Autodesk Fusion 360 part; units mm, degrees
(part 6 of 8)
  spline S180 degree 3 poles (738.6544, -32.0173) (738.4476, -32.017) (738.2428, -32.0571) (737.8602, -32.2135) (737.6859, -32.3284) (737.4231, -32.587) (737.3257, -32.7177) (737.1739, -33.004) (737.1203, -33.1579) (737.0909, -33.3172) knots 0 0 0 0 0.062015 0.062015 0.12403 0.12403 0.172638 0.172638 0.221247 0.221247 0.221247 0.221247
  spline S181 degree 5 poles (738.6544, -32.0173) (738.6823, -32.0173) (738.802, -32.0174) (739.0135, -32.0169) (739.317, -32.0149) (739.7125, -32.0096) (740.1723, -31.9999) (740.6323, -31.9868) (741.0925, -31.9701) (741.553, -31.9499) (742.0138, -31.9262) (742.4748, -31.8993) (742.9359, -31.8692) (743.3973, -31.8361) (743.8588, -31.8) (744.3204, -31.7611) (744.7821, -31.7194) (745.2439, -31.6749) (745.7059, -31.6277) (746.1679, -31.5778) (746.63, -31.5252) (747.0922, -31.47) (747.5544, -31.4123) (748.0167, -31.3521) (748.4791, -31.2893) (748.9414, -31.2242) (749.4038, -31.1567) (749.8663, -31.0868) (750.3287, -31.0146) (750.7911, -30.94) (751.2535, -30.8632) (751.716, -30.7841) (752.1784, -30.7028) (752.6408, -30.6193) (753.1031, -30.5336) (753.5654, -30.4458) (754.0277, -30.3558) (754.4899, -30.2638) (754.9521, -30.1696) (755.4142, -30.0734) (755.8763, -29.9751) (756.3382, -29.8748) (756.8001, -29.7725) (757.262, -29.6682) (757.7237, -29.5619) (758.1854, -29.4537) (758.6469, -29.3435) (759.1084, -29.2314) (759.5698, -29.1173) (760.031, -29.0014) (760.4922, -28.8836) (760.9532, -28.764) (761.4141, -28.6424) (761.8749, -28.5191) (762.3356, -28.3939) (762.7961, -28.2668) (763.2565, -28.138) (763.7168, -28.0074) (764.1769, -27.8751) (764.6368, -27.7409) (765.0966, -27.605) (765.5563, -27.4674) (765.9239, -27.3558) (766.1995, -27.2714) (766.3832, -27.2148) (766.4751, -27.1864) knots 0.13851185 0.13851185 0.13851185 0.13851185 0.13851185 0.13851185 0.14285714 0.15714286 0.17142857 0.18571429 0.2 0.21428571 0.22857143 0.24285714 0.25714286 0.27142857 0.28571429 0.3 0.31428571 0.32857143 0.34285714 0.35714286 0.37142857 0.38571429 0.4 0.41428571 0.42857143 0.44285714 0.45714286 0.47142857 0.48571429 0.5 0.51428571 0.52857143 0.54285714 0.55714286 0.57142857 0.58571429 0.6 0.61428571 0.62857143 0.64285714 0.65714286 0.67142857 0.68571429 0.7 0.71428571 0.72857143 0.74285714 0.75714286 0.77142857 0.78571429 0.8 0.81428571 0.82857143 0.84285714 0.85714286 0.87142857 0.88571429 0.9 0.91428571 0.92857143 0.94285714 0.95714286 0.97142857 0.98571429 1 1 1 1 1 1
  arc A91 (766.4751, -27.1864) -> (767.7563, -17.4547) centre (452.3696, 19.1166) ccw
  spline S182 degree 5 poles (767.7563, -17.4547) (767.6749, -17.4034) (767.5121, -17.3012) (767.2677, -17.1483) (766.9415, -16.9455) (766.5331, -16.6935) (766.1242, -16.4433) (765.7146, -16.1946) (765.3045, -15.9477) (764.8937, -15.7024) (764.4823, -15.4588) (764.0704, -15.217) (763.6578, -14.9768) (763.2446, -14.7384) (762.8309, -14.5017) (762.4165, -14.2668) (762.0016, -14.0336) (761.586, -13.8023) (761.1699, -13.5727) (760.7532, -13.345) (760.3359, -13.1191) (759.918, -12.8951) (759.4994, -12.6729) (759.0803, -12.4526) (758.6607, -12.2343) (758.2404, -12.0178) (757.8195, -11.8033) (757.398, -11.5907) (756.976, -11.3802) (756.5533, -11.1716) (756.1301, -10.9651) (755.7063, -10.7606) (755.2819, -10.5581) (754.8568, -10.3578) (754.4312, -10.1596) (754.005, -9.9635) (753.5783, -9.7696) (753.1509, -9.5779) (752.7229, -9.3885) (752.2943, -9.2013) (751.8652, -9.0164) (751.4354, -8.8338) (751.005, -8.6536) (750.5741, -8.4757) (750.1425, -8.3003) (749.7104, -8.1274) (749.2776, -7.957) (748.8443, -7.7892) (748.4103, -7.624) (747.9757, -7.4616) (747.5405, -7.3018) (747.1047, -7.1447) (746.6683, -6.9904) (746.2312, -6.839) (745.7936, -6.6906) (745.3553, -6.5453) (744.9163, -6.4032) (744.4767, -6.2645) (744.0365, -6.1292) (743.5955, -5.9975) (743.154, -5.8692) (742.7733, -5.7617) (742.4807, -5.6811) (742.2765, -5.626) (742.1608, -5.5951) (742.1339, -5.5879) knots -1 -1 -1 -1 -1 -1 -0.98571429 -0.97142857 -0.95714286 -0.94285714 -0.92857143 -0.91428571 -0.9 -0.88571429 -0.87142857 -0.85714286 -0.84285714 -0.82857143 -0.81428571 -0.8 -0.78571429 -0.77142857 -0.75714286 -0.74285714 -0.72857143 -0.71428571 -0.7 -0.68571429 -0.67142857 -0.65714286 -0.64285714 -0.62857143 -0.61428571 -0.6 -0.58571429 -0.57142857 -0.55714286 -0.54285714 -0.52857143 -0.51428571 -0.5 -0.48571429 -0.47142857 -0.45714286 -0.44285714 -0.42857143 -0.41428571 -0.4 -0.38571429 -0.37142857 -0.35714286 -0.34285714 -0.32857143 -0.31428571 -0.3 -0.28571429 -0.27142857 -0.25714286 -0.24285714 -0.22857143 -0.21428571 -0.2 -0.18571429 -0.17142857 -0.15714286 -0.14285714 -0.13851185 -0.13851185 -0.13851185 -0.13851185 -0.13851185 -0.13851185
  spline S183 degree 3 poles (740.9602, -3.9275) (740.9437, -4.1336) (740.9677, -4.3409) (741.0937, -4.7347) (741.1945, -4.9173) (741.4319, -5.1996) (741.5545, -5.3069) (741.828, -5.4807) (741.9773, -5.5461) (742.1339, -5.5879) knots 0 0 0 0 0.062015 0.062015 0.12403 0.12403 0.172638 0.172638 0.221247 0.221247 0.221247 0.221247
  arc A92 (740.9602, -3.9275) -> (741.4991, 4.2949) centre (452.3696, 19.1166) ccw
  spline S184 degree 3 poles (742.8795, 5.7879) (742.6745, 5.7612) (742.4767, 5.6947) (742.1177, 5.4896) (741.9599, 5.353) (741.7331, 5.0623) (741.6536, 4.92) (741.5404, 4.6163) (741.5074, 4.4567) (741.4991, 4.2949) knots 0 0 0 0 0.062015 0.062015 0.12403 0.12403 0.172638 0.172638 0.221247 0.221247 0.221247 0.221247
  spline S185 degree 5 poles (742.8795, 5.7879) (742.9071, 5.7915) (743.0258, 5.807) (743.2355, 5.8351) (743.5361, 5.8767) (743.9276, 5.9336) (744.3821, 6.0032) (744.8364, 6.0763) (745.2906, 6.1529) (745.7445, 6.233) (746.1983, 6.3166) (746.6518, 6.4035) (747.1051, 6.4935) (747.5582, 6.5866) (748.011, 6.6826) (748.4636, 6.7814) (748.9159, 6.883) (749.368, 6.9874) (749.8198, 7.0945) (750.2713, 7.2043) (750.7226, 7.3167) (751.1737, 7.4318) (751.6244, 7.5493) (752.0749, 7.6694) (752.5251, 7.7919) (752.975, 7.9169) (753.4247, 8.0442) (753.874, 8.1738) (754.323, 8.3058) (754.7718, 8.4401) (755.2202, 8.5766) (755.6684, 8.7153) (756.1162, 8.8563) (756.5637, 8.9995) (757.0109, 9.1448) (757.4578, 9.2922) (757.9044, 9.4417) (758.3507, 9.5933) (758.7966, 9.747) (759.2422, 9.9027) (759.6875, 10.0605) (760.1324, 10.2202) (760.577, 10.3819) (761.0213, 10.5456) (761.4652, 10.7113) (761.9088, 10.8788) (762.352, 11.0483) (762.7949, 11.2197) (763.2374, 11.393) (763.6796, 11.5681) (764.1214, 11.7451) (764.5629, 11.9239) (765.004, 12.1046) (765.4448, 12.287) (765.8851, 12.4713) (766.3252, 12.6573) (766.7648, 12.8451) (767.2041, 13.0347) (767.6429, 13.226) (768.0815, 13.419) (768.5196, 13.6138) (768.9573, 13.8102) (769.3072, 13.9688) (769.5695, 14.0885) (769.7443, 14.1686) (769.8316, 14.2087) knots 0.13851185 0.13851185 0.13851185 0.13851185 0.13851185 0.13851185 0.14285714 0.15714286 0.17142857 0.18571429 0.2 0.21428571 0.22857143 0.24285714 0.25714286 0.27142857 0.28571429 0.3 0.31428571 0.32857143 0.34285714 0.35714286 0.37142857 0.38571429 0.4 0.41428571 0.42857143 0.44285714 0.45714286 0.47142857 0.48571429 0.5 0.51428571 0.52857143 0.54285714 0.55714286 0.57142857 0.58571429 0.6 0.61428571 0.62857143 0.64285714 0.65714286 0.67142857 0.68571429 0.7 0.71428571 0.72857143 0.74285714 0.75714286 0.77142857 0.78571429 0.8 0.81428571 0.82857143 0.84285714 0.85714286 0.87142857 0.88571429 0.9 0.91428571 0.92857143 0.94285714 0.95714286 0.97142857 0.98571429 1 1 1 1 1 1
  arc A93 (769.8316, 14.2087) -> (769.8316, 24.0244) centre (452.3696, 19.1166) ccw
  spline S186 degree 5 poles (769.8316, 24.0244) (769.7443, 24.0646) (769.5695, 24.1447) (769.3072, 24.2644) (768.9573, 24.4229) (768.5196, 24.6194) (768.0815, 24.8142) (767.6429, 25.0072) (767.2041, 25.1985) (766.7648, 25.388) (766.3252, 25.5759) (765.8851, 25.7619) (765.4448, 25.9461) (765.004, 26.1286) (764.5629, 26.3093) (764.1214, 26.4881) (763.6796, 26.6651) (763.2374, 26.8402) (762.7949, 27.0135) (762.352, 27.1848) (761.9088, 27.3543) (761.4652, 27.5219) (761.0213, 27.6875) (760.577, 27.8512) (760.1324, 28.013) (759.6875, 28.1727) (759.2422, 28.3305) (758.7966, 28.4862) (758.3507, 28.6399) (757.9044, 28.7915) (757.4578, 28.941) (757.0109, 29.0884) (756.5637, 29.2337) (756.1162, 29.3769) (755.6684, 29.5178) (755.2202, 29.6566) (754.7718, 29.7931) (754.323, 29.9274) (753.874, 30.0594) (753.4247, 30.189) (752.975, 30.3163) (752.5251, 30.4412) (752.0749, 30.5638) (751.6244, 30.6838) (751.1737, 30.8014) (750.7226, 30.9165) (750.2713, 31.0289) (749.8198, 31.1387) (749.368, 31.2458) (748.9159, 31.3502) (748.4636, 31.4518) (748.011, 31.5506) (747.5582, 31.6466) (747.1051, 31.7397) (746.6518, 31.8297) (746.1983, 31.9166) (745.7445, 32.0001) (745.2906, 32.0803) (744.8364, 32.1569) (744.3821, 32.23) (743.9276, 32.2996) (743.5361, 32.3564) (743.2355, 32.3981) (743.0258, 32.4262) (742.9071, 32.4417) (742.8795, 32.4453) knots -1 -1 -1 -1 -1 -1 -0.98571429 -0.97142857 -0.95714286 -0.94285714 -0.92857143 -0.91428571 -0.9 -0.88571429 -0.87142857 -0.85714286 -0.84285714 -0.82857143 -0.81428571 -0.8 -0.78571429 -0.77142857 -0.75714286 -0.74285714 -0.72857143 -0.71428571 -0.7 -0.68571429 -0.67142857 -0.65714286 -0.64285714 -0.62857143 -0.61428571 -0.6 -0.58571429 -0.57142857 -0.55714286 -0.54285714 -0.52857143 -0.51428571 -0.5 -0.48571429 -0.47142857 -0.45714286 -0.44285714 -0.42857143 -0.41428571 -0.4 -0.38571429 -0.37142857 -0.35714286 -0.34285714 -0.32857143 -0.31428571 -0.3 -0.28571429 -0.27142857 -0.25714286 -0.24285714 -0.22857143 -0.21428571 -0.2 -0.18571429 -0.17142857 -0.15714286 -0.14285714 -0.13851185 -0.13851185 -0.13851185 -0.13851185 -0.13851185 -0.13851185
  spline S187 degree 3 poles (741.4991, 33.9382) (741.5097, 33.7318) (741.5605, 33.5294) (741.7368, 33.1555) (741.8607, 32.9875) (742.1328, 32.7387) (742.2684, 32.6483) (742.5623, 32.5117) (742.7188, 32.4662) (742.8795, 32.4453) knots 0 0 0 0 0.062015 0.062015 0.12403 0.12403 0.172638 0.172638 0.221247 0.221247 0.221247 0.221247
  arc A94 (741.4991, 33.9382) -> (740.9602, 42.1607) centre (452.3696, 19.1166) ccw
  spline S188 degree 3 poles (742.1339, 43.821) (741.9341, 43.7678) (741.7467, 43.6761) (741.4175, 43.4259) (741.2789, 43.2699) (741.092, 42.952) (741.0318, 42.8006) (740.9592, 42.4848) (740.9473, 42.3222) (740.9602, 42.1607) knots 0 0 0 0 0.062015 0.062015 0.12403 0.12403 0.172638 0.172638 0.221247 0.221247 0.221247 0.221247
  spline S189 degree 5 poles (742.1339, 43.821) (742.1608, 43.8282) (742.2765, 43.8591) (742.4807, 43.9143) (742.7733, 43.9949) (743.154, 44.1023) (743.5955, 44.2306) (744.0365, 44.3624) (744.4767, 44.4977) (744.9163, 44.6364) (745.3553, 44.7784) (745.7936, 44.9238) (746.2312, 45.0722) (746.6683, 45.2236) (747.1047, 45.3779) (747.5405, 45.5349) (747.9757, 45.6947) (748.4103, 45.8572) (748.8443, 46.0224) (749.2776, 46.1902) (749.7104, 46.3606) (750.1425, 46.5335) (750.5741, 46.7089) (751.005, 46.8867) (751.4354, 47.067) (751.8652, 47.2496) (752.2943, 47.4345) (752.7229, 47.6217) (753.1509, 47.8111) (753.5783, 48.0028) (754.005, 48.1967) (754.4312, 48.3928) (754.8568, 48.591) (755.2819, 48.7913) (755.7063, 48.9937) (756.1301, 49.1982) (756.5533, 49.4048) (756.976, 49.6133) (757.398, 49.8239) (757.8195, 50.0365) (758.2404, 50.251) (758.6607, 50.4674) (759.0803, 50.6858) (759.4994, 50.9061) (759.918, 51.1283) (760.3359, 51.3523) (760.7532, 51.5782) (761.1699, 51.8059) (761.586, 52.0355) (762.0016, 52.2668) (762.4165, 52.4999) (762.8309, 52.7349) (763.2446, 52.9715) (763.6578, 53.21) (764.0704, 53.4501) (764.4823, 53.692) (764.8937, 53.9356) (765.3045, 54.1809) (765.7146, 54.4278) (766.1242, 54.6764) (766.5331, 54.9267) (766.9415, 55.1786) (767.2677, 55.3815) (767.5121, 55.5344) (767.6749, 55.6366) (767.7563, 55.6878) knots 0.13851185 0.13851185 0.13851185 0.13851185 0.13851185 0.13851185 0.14285714 0.15714286 0.17142857 0.18571429 0.2 0.21428571 0.22857143 0.24285714 0.25714286 0.27142857 0.28571429 0.3 0.31428571 0.32857143 0.34285714 0.35714286 0.37142857 0.38571429 0.4 0.41428571 0.42857143 0.44285714 0.45714286 0.47142857 0.48571429 0.5 0.51428571 0.52857143 0.54285714 0.55714286 0.57142857 0.58571429 0.6 0.61428571 0.62857143 0.64285714 0.65714286 0.67142857 0.68571429 0.7 0.71428571 0.72857143 0.74285714 0.75714286 0.77142857 0.78571429 0.8 0.81428571 0.82857143 0.84285714 0.85714286 0.87142857 0.88571429 0.9 0.91428571 0.92857143 0.94285714 0.95714286 0.97142857 0.98571429 1 1 1 1 1 1
  arc A95 (767.7563, 55.6878) -> (766.4751, 65.4196) centre (452.3696, 19.1166) ccw
  spline S190 degree 5 poles (766.4751, 65.4196) (766.3832, 65.448) (766.1995, 65.5046) (765.9239, 65.589) (765.5563, 65.7005) (765.0966, 65.8382) (764.6368, 65.9741) (764.1769, 66.1082) (763.7168, 66.2406) (763.2565, 66.3712) (762.7961, 66.5) (762.3356, 66.627) (761.8749, 66.7522) (761.4141, 66.8756) (760.9532, 66.9971) (760.4922, 67.1168) (760.031, 67.2346) (759.5698, 67.3505) (759.1084, 67.4645) (758.6469, 67.5766) (758.1854, 67.6868) (757.7237, 67.7951) (757.262, 67.9014) (756.8001, 68.0057) (756.3382, 68.108) (755.8763, 68.2083) (755.4142, 68.3065) (754.9521, 68.4028) (754.4899, 68.4969) (754.0277, 68.589) (753.5654, 68.679) (753.1031, 68.7668) (752.6408, 68.8525) (752.1784, 68.936) (751.716, 69.0173) (751.2535, 69.0964) (750.7911, 69.1732) (750.3287, 69.2477) (749.8663, 69.32) (749.4038, 69.3899) (748.9414, 69.4574) (748.4791, 69.5225) (748.0167, 69.5852) (747.5544, 69.6455) (747.0922, 69.7032) (746.63, 69.7584) (746.1679, 69.811) (745.7059, 69.8609) (745.2439, 69.9081) (744.7821, 69.9526) (744.3204, 69.9943) (743.8588, 70.0332) (743.3973, 70.0692) (742.9359, 70.1024) (742.4748, 70.1325) (742.0138, 70.1594) (741.553, 70.183) (741.0925, 70.2032) (740.6323, 70.2199) (740.1723, 70.2331) (739.7125, 70.2428) (739.317, 70.248) (739.0135, 70.2501) (738.802, 70.2506) (738.6823, 70.2505) (738.6544, 70.2504) knots -1 -1 -1 -1 -1 -1 -0.98571429 -0.97142857 -0.95714286 -0.94285714 -0.92857143 -0.91428571 -0.9 -0.88571429 -0.87142857 -0.85714286 -0.84285714 -0.82857143 -0.81428571 -0.8 -0.78571429 -0.77142857 -0.75714286 -0.74285714 -0.72857143 -0.71428571 -0.7 -0.68571429 -0.67142857 -0.65714286 -0.64285714 -0.62857143 -0.61428571 -0.6 -0.58571429 -0.57142857 -0.55714286 -0.54285714 -0.52857143 -0.51428571 -0.5 -0.48571429 -0.47142857 -0.45714286 -0.44285714 -0.42857143 -0.41428571 -0.4 -0.38571429 -0.37142857 -0.35714286 -0.34285714 -0.32857143 -0.31428571 -0.3 -0.28571429 -0.27142857 -0.25714286 -0.24285714 -0.22857143 -0.21428571 -0.2 -0.18571429 -0.17142857 -0.15714286 -0.14285714 -0.13851185 -0.13851185 -0.13851185 -0.13851185 -0.13851185 -0.13851185
  spline S191 degree 3 poles (737.0909, 71.5504) (737.1284, 71.3471) (737.2052, 71.1531) (737.4288, 70.8054) (737.5735, 70.655) (737.8758, 70.4438) (738.022, 70.3719) (738.3312, 70.2748) (738.4923, 70.2502) (738.6544, 70.2504) knots 0 0 0 0 0.062015 0.062015 0.12403 0.12403 0.172638 0.172638 0.221247 0.221247 0.221247 0.221247
  circle A96 centre (452.3696, 19.1166) radius 12.7
  circle A97 centre (452.3696, 19.1166) radius 12.7
  dimension "d17" = 25.4
  constraint concentric A0 A97
  measures "d17" diameter of A97
extrude "Extrude1''" add sketch "Sketch1 (3)" along normal mid plane 152.4 separate body contours A96 A97 makes body 3 in component "Component"
sketch "Sketch2 (3)" plane through (0, 0, 12.7) normal (0, 0, 1) x (1, 0, 0)
  arc A0 (126.3672, -24.5983) -> (127.7662, -13.9721) centre (-8.7656, -1.4025) ccw
  arc A1 (129.4742, -12.5352) -> (127.7662, -13.9721) centre (129.347, -14.1176) ccw
  line L0 (129.4742, -12.5352) -> (133.9814, -12.8976)
  spline S0 degree 5 poles (133.9814, -12.8976) (134.0461, -12.9028) (134.1756, -12.9115) (134.3698, -12.9198) (134.629, -12.9214) (134.9532, -12.9107) (135.2776, -12.8908) (135.6022, -12.8653) (135.9267, -12.8368) (136.2513, -12.8063) (136.5759, -12.7736) (136.9004, -12.738) (137.2248, -12.6986) (137.5492, -12.6547) (137.8735, -12.6064) (138.1976, -12.5541) (138.5217, -12.4982) (138.8456, -12.4395) (139.1694, -12.3782) (139.493, -12.3146) (139.8164, -12.2485) (140.1397, -12.1799) (140.4628, -12.1087) (140.7857, -12.0347) (141.1085, -11.958) (141.431, -11.8787) (141.7533, -11.797) (142.0754, -11.713) (142.3973, -11.6267) (142.719, -11.5383) (143.0404, -11.4476) (143.3616, -11.3548) (143.6826, -11.2599) (144.0033, -11.1627) (144.3237, -11.0635) (144.6439, -10.9621) (144.9639, -10.8587) (145.2835, -10.7533) (145.6029, -10.6459) (145.922, -10.5366) (146.2409, -10.4253) (146.5594, -10.3121) (146.8777, -10.1971) (147.1957, -10.0801) (147.5133, -9.9613) (147.8307, -9.8407) (148.1478, -9.7182) (148.4645, -9.5939) (148.781, -9.4679) (149.0971, -9.3401) (149.4129, -9.2105) (149.7284, -9.0792) (150.0435, -8.9462) (150.3583, -8.8115) (150.6728, -8.6752) (150.9869, -8.5371) (151.3007, -8.3974) (151.6142, -8.256) (151.9273, -8.113) (152.24, -7.9684) (152.5524, -7.8221) (152.8644, -7.6743) (153.1761, -7.5249) (153.4874, -7.3739) (153.7983, -7.2214) (154.1088, -7.0673) (154.419, -6.9116) (154.7288, -6.7545) (155.0382, -6.5958) (155.3472, -6.4356) (155.6559, -6.2739) (155.9024, -6.1434) (156.0872, -6.0448) (156.2103, -5.9788) (156.2719, -5.9457) knots 0 0 0 0 0 0 0.01428571 0.02857143 0.04285714 0.05714286 0.07142857 0.08571429 0.1 0.11428571 0.12857143 0.14285714 0.15714286 0.17142857 0.18571429 0.2 0.21428571 0.22857143 0.24285714 0.25714286 0.27142857 0.28571429 0.3 0.31428571 0.32857143 0.34285714 0.35714286 0.37142857 0.38571429 0.4 0.41428571 0.42857143 0.44285714 0.45714286 0.47142857 0.48571429 0.5 0.51428571 0.52857143 0.54285714 0.55714286 0.57142857 0.58571429 0.6 0.61428571 0.62857143 0.64285714 0.65714286 0.67142857 0.68571429 0.7 0.71428571 0.72857143 0.74285714 0.75714286 0.77142857 0.78571429 0.8 0.81428571 0.82857143 0.84285714 0.85714286 0.87142857 0.88571429 0.9 0.91428571 0.92857143 0.94285714 0.95714286 0.97142857 0.98571429 1 1 1 1 1 1
  arc A2 (156.2719, -5.9457) -> (156.2719, 3.1407) centre (-8.7656, -1.4025) ccw
  spline S1 degree 5 poles (156.2719, 3.1407) (156.2103, 3.1738) (156.0872, 3.2398) (155.9024, 3.3384) (155.6559, 3.4689) (155.3472, 3.6306) (155.0382, 3.7908) (154.7288, 3.9495) (154.419, 4.1066) (154.1088, 4.2623) (153.7983, 4.4164) (153.4874, 4.5689) (153.1761, 4.7199) (152.8644, 4.8693) (152.5524, 5.0171) (152.24, 5.1634) (151.9273, 5.308) (151.6142, 5.451) (151.3007, 5.5924) (150.9869, 5.7321) (150.6728, 5.8702) (150.3583, 6.0065) (150.0435, 6.1412) (149.7284, 6.2742) (149.4129, 6.4055) (149.0971, 6.5351) (148.781, 6.6629) (148.4645, 6.7889) (148.1478, 6.9132) (147.8307, 7.0357) (147.5133, 7.1563) (147.1957, 7.2751) (146.8777, 7.3921) (146.5594, 7.5071) (146.2409, 7.6203) (145.922, 7.7316) (145.6029, 7.8409) (145.2835, 7.9483) (144.9639, 8.0537) (144.6439, 8.1571) (144.3237, 8.2585) (144.0033, 8.3577) (143.6826, 8.4549) (143.3616, 8.5498) (143.0404, 8.6426) (142.719, 8.7333) (142.3973, 8.8217) (142.0754, 8.908) (141.7533, 8.992) (141.431, 9.0737) (141.1085, 9.153) (140.7857, 9.2297) (140.4628, 9.3037) (140.1397, 9.3749) (139.8164, 9.4435) (139.493, 9.5096) (139.1694, 9.5732) (138.8456, 9.6345) (138.5217, 9.6932) (138.1976, 9.7491) (137.8735, 9.8014) (137.5492, 9.8497) (137.2248, 9.8936) (136.9004, 9.933) (136.5759, 9.9686) (136.2513, 10.0013) (135.9267, 10.0318) (135.6022, 10.0603) (135.2776, 10.0858) (134.9532, 10.1057) (134.629, 10.1164) (134.3698, 10.1148) (134.1756, 10.1065) (134.0461, 10.0978) (133.9814, 10.0926) knots -1 -1 -1 -1 -1 -1 -0.98571429 -0.97142857 -0.95714286 -0.94285714 -0.92857143 -0.91428571 -0.9 -0.88571429 -0.87142857 -0.85714286 -0.84285714 -0.82857143 -0.81428571 -0.8 -0.78571429 -0.77142857 -0.75714286 -0.74285714 -0.72857143 -0.71428571 -0.7 -0.68571429 -0.67142857 -0.65714286 -0.64285714 -0.62857143 -0.61428571 -0.6 -0.58571429 -0.57142857 -0.55714286 -0.54285714 -0.52857143 -0.51428571 -0.5 -0.48571429 -0.47142857 -0.45714286 -0.44285714 -0.42857143 -0.41428571 -0.4 -0.38571429 -0.37142857 -0.35714286 -0.34285714 -0.32857143 -0.31428571 -0.3 -0.28571429 -0.27142857 -0.25714286 -0.24285714 -0.22857143 -0.21428571 -0.2 -0.18571429 -0.17142857 -0.15714286 -0.14285714 -0.12857143 -0.11428571 -0.1 -0.08571429 -0.07142857 -0.05714286 -0.04285714 -0.02857143 -0.01428571 0 0 0 0 0 0
  line L1 (133.9814, 10.0926) -> (129.4742, 9.7302)
  arc A3 (127.7662, 11.1671) -> (129.4742, 9.7302) centre (129.347, 11.3126) ccw
  arc A4 (127.7662, 11.1671) -> (126.3672, 21.7933) centre (-8.7656, -1.4025) ccw
  arc A5 (127.6452, 23.6232) -> (126.3672, 21.7933) centre (127.9319, 22.0618) ccw
  line L2 (127.6452, 23.6232) -> (132.0926, 24.4398)
  spline S2 degree 5 poles (132.0926, 24.4398) (132.1564, 24.4515) (132.2837, 24.4765) (132.4735, 24.5188) (132.7242, 24.5844) (133.0346, 24.6786) (133.3429, 24.7818) (133.6497, 24.8904) (133.9559, 25.0019) (134.2615, 25.1154) (134.5666, 25.231) (134.8708, 25.3494) (135.174, 25.4714) (135.4759, 25.5977) (135.7767, 25.7283) (136.0762, 25.8628) (136.3748, 26.0006) (136.6724, 26.1412) (136.9693, 26.2842) (137.2655, 26.4294) (137.5608, 26.5769) (137.8553, 26.7268) (138.149, 26.8793) (138.4417, 27.0343) (138.7336, 27.1919) (139.0246, 27.352) (139.3148, 27.5143) (139.6042, 27.6789) (139.8928, 27.8455) (140.1806, 28.0142) (140.4676, 28.1849) (140.7539, 28.3577) (141.0393, 28.5325) (141.3239, 28.7093) (141.6078, 28.8882) (141.8908, 29.0689) (142.1731, 29.2516) (142.4546, 29.4362) (142.7353, 29.6226) (143.0153, 29.8108) (143.2944, 30.0008) (143.5728, 30.1925) (143.8505, 30.386) (144.1273, 30.5813) (144.4034, 30.7783) (144.6788, 30.977) (144.9533, 31.1773) (145.2271, 31.3793) (145.5002, 31.583) (145.7724, 31.7883) (146.0439, 31.9951) (146.3147, 32.2036) (146.5847, 32.4136) (146.8539, 32.6252) (147.1224, 32.8384) (147.3901, 33.053) (147.657, 33.2692) (147.9232, 33.4869) (148.1886, 33.706) (148.4532, 33.9267) (148.7171, 34.1488) (148.9803, 34.3723) (149.2426, 34.5973) (149.5042, 34.8237) (149.7651, 35.0515) (150.0252, 35.2808) (150.2845, 35.5114) (150.5431, 35.7434) (150.8009, 35.9767) (151.0579, 36.2114) (151.3141, 36.4475) (151.5185, 36.6374) (151.6715, 36.7805) (151.7733, 36.8761) (151.8242, 36.924) knots 0 0 0 0 0 0 0.01428571 0.02857143 0.04285714 0.05714286 0.07142857 0.08571429 0.1 0.11428571 0.12857143 0.14285714 0.15714286 0.17142857 0.18571429 0.2 0.21428571 0.22857143 0.24285714 0.25714286 0.27142857 0.28571429 0.3 0.31428571 0.32857143 0.34285714 0.35714286 0.37142857 0.38571429 0.4 0.41428571 0.42857143 0.44285714 0.45714286 0.47142857 0.48571429 0.5 0.51428571 0.52857143 0.54285714 0.55714286 0.57142857 0.58571429 0.6 0.61428571 0.62857143 0.64285714 0.65714286 0.67142857 0.68571429 0.7 0.71428571 0.72857143 0.74285714 0.75714286 0.77142857 0.78571429 0.8 0.81428571 0.82857143 0.84285714 0.85714286 0.87142857 0.88571429 0.9 0.91428571 0.92857143 0.94285714 0.95714286 0.97142857 0.98571429 1 1 1 1 1 1
  arc A6 (151.8242, 36.924) -> (149.4725, 45.7007) centre (-8.7656, -1.4025) ccw
  spline S3 degree 5 poles (149.4725, 45.7007) (149.4045, 45.7167) (149.2685, 45.7487) (149.0645, 45.7961) (148.7925, 45.8583) (148.4525, 45.9346) (148.1126, 46.0094) (147.7727, 46.0826) (147.4328, 46.1542) (147.0929, 46.2243) (146.753, 46.2927) (146.4132, 46.3596) (146.0734, 46.4249) (145.7337, 46.4885) (145.3941, 46.5506) (145.0545, 46.611) (144.715, 46.6697) (144.3755, 46.7268) (144.0362, 46.7822) (143.6969, 46.836) (143.3578, 46.888) (143.0187, 46.9384) (142.6797, 46.987) (142.3409, 47.0339) (142.0022, 47.0791) (141.6636, 47.1225) (141.3252, 47.1641) (140.9869, 47.204) (140.6488, 47.242) (140.3109, 47.2783) (139.9731, 47.3127) (139.6355, 47.3452) (139.2981, 47.3759) (138.9609, 47.4046) (138.6239, 47.4315) (138.2871, 47.4565) (137.9506, 47.4795) (137.6143, 47.5005) (137.2782, 47.5196) (136.9424, 47.5367) (136.6069, 47.5517) (136.2717, 47.5647) (135.9367, 47.5755) (135.6022, 47.5841) (135.2679, 47.5906) (134.9339, 47.595) (134.6004, 47.5972) (134.2671, 47.5972) (133.9342, 47.595) (133.6017, 47.5905) (133.2697, 47.5836) (132.9381, 47.5742) (132.607, 47.5621) (132.2765, 47.5473) (131.9465, 47.5298) (131.6169, 47.5099) (131.2879, 47.4876) (130.9593, 47.463) (130.6312, 47.4359) (130.3037, 47.406) (129.9771, 47.3727) (129.6513, 47.3354) (129.3267, 47.2938) (129.0031, 47.2479) (128.6804, 47.1983) (128.3585, 47.1459) (128.037, 47.0914) (127.7162, 47.0349) (127.3961, 46.9755) (127.0776, 46.9107) (126.7616, 46.8371) (126.5117, 46.7685) (126.3262, 46.7103) (126.2035, 46.6683) (126.1423, 46.6466) knots -1 -1 -1 -1 -1 -1 -0.98571429 -0.97142857 -0.95714286 -0.94285714 -0.92857143 -0.91428571 -0.9 -0.88571429 -0.87142857 -0.85714286 -0.84285714 -0.82857143 -0.81428571 -0.8 -0.78571429 -0.77142857 -0.75714286 -0.74285714 -0.72857143 -0.71428571 -0.7 -0.68571429 -0.67142857 -0.65714286 -0.64285714 -0.62857143 -0.61428571 -0.6 -0.58571429 -0.57142857 -0.55714286 -0.54285714 -0.52857143 -0.51428571 -0.5 -0.48571429 -0.47142857 -0.45714286 -0.44285714 -0.42857143 -0.41428571 -0.4 -0.38571429 -0.37142857 -0.35714286 -0.34285714 -0.32857143 -0.31428571 -0.3 -0.28571429 -0.27142857 -0.25714286 -0.24285714 -0.22857143 -0.21428571 -0.2 -0.18571429 -0.17142857 -0.15714286 -0.14285714 -0.12857143 -0.11428571 -0.1 -0.08571429 -0.07142857 -0.05714286 -0.04285714 -0.02857143 -0.01428571 0 0 0 0 0 0
  line L3 (126.1423, 46.6466) -> (121.8825, 45.13)
  arc A7 (119.8607, 46.0758) -> (121.8825, 45.13) centre (121.35, 46.6255) ccw
  arc A8 (119.8607, 46.0758) -> (115.7592, 55.9778) centre (-8.7656, -1.4025) ccw
  arc A9 (116.52, 58.0762) -> (115.7592, 55.9778) centre (117.201, 56.6422) ccw
  line L4 (116.52, 58.0762) -> (120.6045, 60.016)
  spline S4 degree 5 poles (120.6045, 60.016) (120.6631, 60.0438) (120.7796, 60.101) (120.9519, 60.191) (121.1772, 60.3192) (121.4526, 60.4906) (121.7236, 60.67) (121.992, 60.8543) (122.2588, 61.0413) (122.5246, 61.23) (122.7894, 61.4206) (123.0526, 61.6137) (123.3139, 61.81) (123.5728, 62.0102) (123.8295, 62.2141) (124.0841, 62.4216) (124.3368, 62.632) (124.5879, 62.8448) (124.8377, 63.0598) (125.0861, 63.2767) (125.3332, 63.4956) (125.5789, 63.7166) (125.8231, 63.9399) (126.0658, 64.1654) (126.3069, 64.3932) (126.5466, 64.6231) (126.7849, 64.8551) (127.0218, 65.0889) (127.2574, 65.3245) (127.4918, 65.562) (127.7248, 65.8012) (127.9566, 66.0421) (128.1871, 66.2849) (128.4162, 66.5293) (128.6441, 66.7755) (128.8707, 67.0234) (129.0961, 67.2729) (129.3202, 67.524) (129.5432, 67.7767) (129.7649, 68.031) (129.9854, 68.2868) (130.2046, 68.544) (130.4227, 68.8028) (130.6396, 69.0631) (130.8553, 69.3248) (131.0699, 69.588) (131.2832, 69.8526) (131.4954, 70.1186) (131.7064, 70.386) (131.9163, 70.6547) (132.125, 70.9248) (132.3326, 71.1962) (132.539, 71.469) (132.7443, 71.743) (132.9484, 72.0184) (133.1514, 72.295) (133.3533, 72.5729) (133.5541, 72.8521) (133.7537, 73.1325) (133.9523, 73.4141) (134.1497, 73.6969) (134.346, 73.981) (134.5412, 74.2662) (134.7353, 74.5526) (134.9283, 74.8402) (135.1202, 75.1289) (135.311, 75.4188) (135.5007, 75.7098) (135.6893, 76.0019) (135.8768, 76.2951) (136.0633, 76.5895) (136.2115, 76.8258) (136.3223, 77.0036) (136.3959, 77.1223) (136.4326, 77.1817) knots 0 0 0 0 0 0 0.01428571 0.02857143 0.04285714 0.05714286 0.07142857 0.08571429 0.1 0.11428571 0.12857143 0.14285714 0.15714286 0.17142857 0.18571429 0.2 0.21428571 0.22857143 0.24285714 0.25714286 0.27142857 0.28571429 0.3 0.31428571 0.32857143 0.34285714 0.35714286 0.37142857 0.38571429 0.4 0.41428571 0.42857143 0.44285714 0.45714286 0.47142857 0.48571429 0.5 0.51428571 0.52857143 0.54285714 0.55714286 0.57142857 0.58571429 0.6 0.61428571 0.62857143 0.64285714 0.65714286 0.67142857 0.68571429 0.7 0.71428571 0.72857143 0.74285714 0.75714286 0.77142857 0.78571429 0.8 0.81428571 0.82857143 0.84285714 0.85714286 0.87142857 0.88571429 0.9 0.91428571 0.92857143 0.94285714 0.95714286 0.97142857 0.98571429 1 1 1 1 1 1
  arc A10 (136.4326, 77.1817) -> (131.8894, 85.0507) centre (-8.7656, -1.4025) ccw
  spline S5 degree 5 poles (131.8894, 85.0507) (131.8196, 85.0486) (131.68, 85.0443) (131.4707, 85.0372) (131.1918, 85.027) (130.8437, 85.0127) (130.496, 84.9969) (130.1487, 84.9797) (129.8019, 84.9609) (129.4554, 84.9406) (129.1094, 84.9187) (128.7639, 84.8954) (128.4188, 84.8705) (128.0742, 84.8441) (127.73, 84.8161) (127.3864, 84.7865) (127.0432, 84.7554) (126.7006, 84.7227) (126.3585, 84.6884) (126.0169, 84.6525) (125.6758, 84.615) (125.3352, 84.5759) (124.9952, 84.5351) (124.6558, 84.4927) (124.317, 84.4487) (123.9787, 84.403) (123.641, 84.3556) (123.304, 84.3066) (122.9675, 84.2558) (122.6317, 84.2033) (122.2965, 84.1491) (121.962, 84.0932) (121.6282, 84.0355) (121.295, 83.976) (120.9625, 83.9147) (120.6308, 83.8517) (120.2998, 83.7868) (119.9695, 83.7201) (119.6399, 83.6516) (119.3111, 83.5811) (118.9832, 83.5088) (118.656, 83.4346) (118.3297, 83.3583) (118.0043, 83.2801) (117.6797, 83.1999) (117.356, 83.1176) (117.0332, 83.0334) (116.7113, 82.9472) (116.3904, 82.8589) (116.0704, 82.7685) (115.7514, 82.6759) (115.4336, 82.5809) (115.1169, 82.4836) (114.8015, 82.3837) (114.4872, 82.2815) (114.1741, 82.1769) (113.862, 82.0702) (113.551, 81.9614) (113.2411, 81.8503) (112.9325, 81.7367) (112.6256, 81.6199) (112.3206, 81.4996) (112.0178, 81.3754) (111.7171, 81.2474) (111.4183, 81.1159) (111.1208, 80.982) (110.8245, 80.8461) (110.5291, 80.7085) (110.2354, 80.5683) (109.9445, 80.4233) (109.6583, 80.2704) (109.4347, 80.1395) (109.2706, 80.0352) (109.1629, 79.9629) (109.1094, 79.9261) knots -1 -1 -1 -1 -1 -1 -0.98571429 -0.97142857 -0.95714286 -0.94285714 -0.92857143 -0.91428571 -0.9 -0.88571429 -0.87142857 -0.85714286 -0.84285714 -0.82857143 -0.81428571 -0.8 -0.78571429 -0.77142857 -0.75714286 -0.74285714 -0.72857143 -0.71428571 -0.7 -0.68571429 -0.67142857 -0.65714286 -0.64285714 -0.62857143 -0.61428571 -0.6 -0.58571429 -0.57142857 -0.55714286 -0.54285714 -0.52857143 -0.51428571 -0.5 -0.48571429 -0.47142857 -0.45714286 -0.44285714 -0.42857143 -0.41428571 -0.4 -0.38571429 -0.37142857 -0.35714286 -0.34285714 -0.32857143 -0.31428571 -0.3 -0.28571429 -0.27142857 -0.25714286 -0.24285714 -0.22857143 -0.21428571 -0.2 -0.18571429 -0.17142857 -0.15714286 -0.14285714 -0.12857143 -0.11428571 -0.1 -0.08571429 -0.07142857 -0.05714286 -0.04285714 -0.02857143 -0.01428571 0 0 0 0 0 0
  line L5 (109.1094, 79.9261) -> (105.3872, 77.3586)
  arc A11 (103.1896, 77.749) -> (105.3872, 77.3586) centre (104.4859, 78.6654) ccw
  arc A12 (103.1896, 77.749) -> (96.665, 86.252) centre (-8.7656, -1.4025) ccw
  arc A13 (96.8567, 88.4758) -> (96.665, 86.252) centre (97.8857, 87.2669) ccw
  line L6 (96.8567, 88.4758) -> (100.3, 91.4067)
  spline S6 degree 5 poles (100.3, 91.4067) (100.3495, 91.4487) (100.4472, 91.5341) (100.5904, 91.6656) (100.7748, 91.8477) (100.9964, 92.0846) (101.2118, 92.328) (101.4232, 92.5755) (101.6326, 92.8252) (101.8405, 93.0763) (102.0469, 93.3289) (102.2512, 93.5835) (102.4528, 93.8408) (102.6511, 94.1012) (102.8463, 94.3646) (103.0385, 94.6309) (103.2281, 94.8995) (103.4156, 95.1701) (103.6012, 95.4423) (103.785, 95.7162) (103.9671, 95.9916) (104.1472, 96.2687) (104.3252, 96.5475) (104.5013, 96.8282) (104.6752, 97.1106) (104.8473, 97.3947) (105.0174, 97.6804) (105.1857, 97.9676) (105.3523, 98.2562) (105.5172, 98.5462) (105.6804, 98.8376) (105.8419, 99.1303) (106.0017, 99.4244) (106.1598, 99.7199) (106.3162, 100.0167) (106.471, 100.3148) (106.6241, 100.6141) (106.7756, 100.9147) (106.9255, 101.2165) (107.0738, 101.5194) (107.2206, 101.8235) (107.3658, 102.1288) (107.5095, 102.4352) (107.6517, 102.7428) (107.7923, 103.0514) (107.9314, 103.3611) (108.069, 103.6719) (108.2051, 103.9838) (108.3397, 104.2967) (108.4729, 104.6106) (108.6046, 104.9255) (108.7348, 105.2414) (108.8636, 105.5583) (108.991, 105.8761) (109.1169, 106.1949) (109.2414, 106.5147) (109.3645, 106.8354) (109.4862, 107.157) (109.6064, 107.4795) (109.7253, 107.8029) (109.8428, 108.1272) (109.9589, 108.4523) (110.0736, 108.7784) (110.187, 109.1053) (110.299, 109.433) (110.4096, 109.7615) (110.5189, 110.0909) (110.6268, 110.4211) (110.7334, 110.7521) (110.8386, 111.0839) (110.9425, 111.4164) (111.0246, 111.6831) (111.0855, 111.8835) (111.1259, 112.0172) (111.146, 112.0841) knots 0 0 0 0 0 0 0.01428571 0.02857143 0.04285714 0.05714286 0.07142857 0.08571429 0.1 0.11428571 0.12857143 0.14285714 0.15714286 0.17142857 0.18571429 0.2 0.21428571 0.22857143 0.24285714 0.25714286 0.27142857 0.28571429 0.3 0.31428571 0.32857143 0.34285714 0.35714286 0.37142857 0.38571429 0.4 0.41428571 0.42857143 0.44285714 0.45714286 0.47142857 0.48571429 0.5 0.51428571 0.52857143 0.54285714 0.55714286 0.57142857 0.58571429 0.6 0.61428571 0.62857143 0.64285714 0.65714286 0.67142857 0.68571429 0.7 0.71428571 0.72857143 0.74285714 0.75714286 0.77142857 0.78571429 0.8 0.81428571 0.82857143 0.84285714 0.85714286 0.87142857 0.88571429 0.9 0.91428571 0.92857143 0.94285714 0.95714286 0.97142857 0.98571429 1 1 1 1 1 1
  arc A14 (111.146, 112.0841) -> (104.721, 118.5091) centre (-8.7656, -1.4025) ccw
  spline S7 degree 5 poles (104.721, 118.5091) (104.6541, 118.489) (104.5204, 118.4487) (104.32, 118.3877) (104.0533, 118.3057) (103.7207, 118.2018) (103.389, 118.0965) (103.058, 117.9899) (102.7278, 117.882) (102.3984, 117.7727) (102.0699, 117.6621) (101.7421, 117.5501) (101.4153, 117.4368) (101.0892, 117.322) (100.7641, 117.2059) (100.4398, 117.0884) (100.1164, 116.9696) (99.7939, 116.8493) (99.4723, 116.7276) (99.1516, 116.6045) (98.8318, 116.48) (98.513, 116.3541) (98.1952, 116.2267) (97.8783, 116.0979) (97.5624, 115.9677) (97.2475, 115.836) (96.9335, 115.7028) (96.6207, 115.5682) (96.3088, 115.4321) (95.998, 115.2945) (95.6883, 115.1554) (95.3797, 115.0148) (95.0721, 114.8726) (94.7657, 114.729) (94.4604, 114.5837) (94.1563, 114.437) (93.8533, 114.2886) (93.5516, 114.1387) (93.251, 113.9872) (92.9516, 113.8341) (92.6536, 113.6794) (92.3568, 113.5229) (92.0613, 113.3649) (91.7672, 113.2051) (91.4745, 113.0436) (91.1831, 112.8804) (90.8931, 112.7154) (90.6045, 112.5488) (90.3173, 112.3805) (90.0316, 112.2104) (89.7475, 112.0384) (89.4651, 111.8644) (89.1844, 111.6884) (88.9056, 111.5103) (88.6285, 111.3302) (88.353, 111.1482) (88.0792, 110.9643) (87.807, 110.7787) (87.5364, 110.5912) (87.2677, 110.4016) (87.0015, 110.2094) (86.738, 110.0142) (86.4777, 109.8159) (86.2204, 109.6143) (85.9658, 109.4101) (85.7131, 109.2037) (85.462, 108.9957) (85.2124, 108.7864) (84.9649, 108.5749) (84.7214, 108.3596) (84.4846, 108.1379) (84.3025, 107.9535) (84.1709, 107.8103) (84.0856, 107.7126) (84.0435, 107.6632) knots -1 -1 -1 -1 -1 -1 -0.98571429 -0.97142857 -0.95714286 -0.94285714 -0.92857143 -0.91428571 -0.9 -0.88571429 -0.87142857 -0.85714286 -0.84285714 -0.82857143 -0.81428571 -0.8 -0.78571429 -0.77142857 -0.75714286 -0.74285714 -0.72857143 -0.71428571 -0.7 -0.68571429 -0.67142857 -0.65714286 -0.64285714 -0.62857143 -0.61428571 -0.6 -0.58571429 -0.57142857 -0.55714286 -0.54285714 -0.52857143 -0.51428571 -0.5 -0.48571429 -0.47142857 -0.45714286 -0.44285714 -0.42857143 -0.41428571 -0.4 -0.38571429 -0.37142857 -0.35714286 -0.34285714 -0.32857143 -0.31428571 -0.3 -0.28571429 -0.27142857 -0.25714286 -0.24285714 -0.22857143 -0.21428571 -0.2 -0.18571429 -0.17142857 -0.15714286 -0.14285714 -0.12857143 -0.11428571 -0.1 -0.08571429 -0.07142857 -0.05714286 -0.04285714 -0.02857143 -0.01428571 0 0 0 0 0 0
  line L7 (84.0435, 107.6632) -> (81.1127, 104.2199)
  arc A15 (78.8889, 104.0281) -> (81.1127, 104.2199) centre (79.9038, 105.2488) ccw
  arc A16 (78.8889, 104.0281) -> (70.3859, 110.5527) centre (-8.7656, -1.4025) ccw
  arc A17 (69.9955, 112.7504) -> (70.3859, 110.5527) centre (71.3023, 111.849) ccw
  line L8 (69.9955, 112.7504) -> (72.5629, 116.4725)
  spline S8 degree 5 poles (72.5629, 116.4725) (72.5998, 116.526) (72.6721, 116.6337) (72.7763, 116.7978) (72.9073, 117.0214) (73.0602, 117.3076) (73.2052, 117.5985) (73.3454, 117.8923) (73.483, 118.1876) (73.6188, 118.484) (73.7528, 118.7814) (73.8842, 119.0802) (74.0123, 119.3809) (74.1365, 119.6837) (74.2568, 119.9887) (74.3736, 120.2956) (74.4872, 120.6042) (74.5983, 120.9141) (74.7071, 121.2251) (74.8138, 121.5372) (74.9183, 121.8503) (75.0206, 122.1646) (75.1204, 122.48) (75.2178, 122.7967) (75.3128, 123.1145) (75.4054, 123.4335) (75.4958, 123.7535) (75.584, 124.0744) (75.6703, 124.3963) (75.7545, 124.7191) (75.8367, 125.0428) (75.917, 125.3674) (75.9952, 125.6928) (76.0714, 126.0191) (76.1457, 126.3463) (76.218, 126.6743) (76.2884, 127.003) (76.357, 127.3326) (76.4237, 127.6629) (76.4886, 127.9939) (76.5516, 128.3257) (76.6129, 128.6581) (76.6724, 128.9913) (76.7301, 129.3251) (76.786, 129.6596) (76.8402, 129.9948) (76.8927, 130.3306) (76.9434, 130.6671) (76.9925, 131.0041) (77.0399, 131.3418) (77.0856, 131.6801) (77.1296, 132.0189) (77.172, 132.3584) (77.2128, 132.6983) (77.2519, 133.0389) (77.2894, 133.38) (77.3253, 133.7216) (77.3596, 134.0637) (77.3923, 134.4064) (77.4234, 134.7495) (77.453, 135.0932) (77.4809, 135.4373) (77.5074, 135.7819) (77.5323, 136.127) (77.5556, 136.4725) (77.5774, 136.8185) (77.5977, 137.165) (77.6165, 137.5118) (77.6338, 137.8591) (77.6496, 138.2068) (77.6639, 138.555) (77.6741, 138.8338) (77.6811, 139.0431) (77.6855, 139.1827) (77.6876, 139.2526) knots 0 0 0 0 0 0 0.01428571 0.02857143 0.04285714 0.05714286 0.07142857 0.08571429 0.1 0.11428571 0.12857143 0.14285714 0.15714286 0.17142857 0.18571429 0.2 0.21428571 0.22857143 0.24285714 0.25714286 0.27142857 0.28571429 0.3 0.31428571 0.32857143 0.34285714 0.35714286 0.37142857 0.38571429 0.4 0.41428571 0.42857143 0.44285714 0.45714286 0.47142857 0.48571429 0.5 0.51428571 0.52857143 0.54285714 0.55714286 0.57142857 0.58571429 0.6 0.61428571 0.62857143 0.64285714 0.65714286 0.67142857 0.68571429 0.7 0.71428571 0.72857143 0.74285714 0.75714286 0.77142857 0.78571429 0.8 0.81428571 0.82857143 0.84285714 0.85714286 0.87142857 0.88571429 0.9 0.91428571 0.92857143 0.94285714 0.95714286 0.97142857 0.98571429 1 1 1 1 1 1
  arc A18 (77.6876, 139.2526) -> (69.8186, 143.7957) centre (-8.7656, -1.4025) ccw
  spline S9 degree 5 poles (69.8186, 143.7957) (69.7592, 143.759) (69.6405, 143.6854) (69.4627, 143.5747) (69.2263, 143.4264) (68.932, 143.2399) (68.6388, 143.0524) (68.3466, 142.8638) (68.0556, 142.6741) (67.7658, 142.4833) (67.477, 142.2914) (67.1895, 142.0984) (66.9031, 141.9043) (66.6178, 141.7091) (66.3338, 141.5128) (66.051, 141.3154) (65.7694, 141.1169) (65.489, 140.9172) (65.2098, 140.7165) (64.9319, 140.5146) (64.6553, 140.3115) (64.3799, 140.1074) (64.1059, 139.9021) (63.8331, 139.6957) (63.5617, 139.4881) (63.2916, 139.2794) (63.0228, 139.0695) (62.7555, 138.8585) (62.4895, 138.6463) (62.2249, 138.433) (61.9617, 138.2185) (61.7, 138.0027) (61.4397, 137.7859) (61.1809, 137.5678) (60.9236, 137.3485) (60.6679, 137.128) (60.4136, 136.9063) (60.1609, 136.6834) (59.9098, 136.4592) (59.6603, 136.2339) (59.4124, 136.0072) (59.1662, 135.7794) (58.9217, 135.5502) (58.679, 135.3197) (58.4381, 135.088) (58.1989, 134.8549) (57.9614, 134.6206) (57.7258, 134.3849) (57.4919, 134.148) (57.26, 133.9097) (57.0301, 133.67) (56.8023, 133.4289) (56.5768, 133.1862) (56.3535, 132.942) (56.1325, 132.6964) (55.9136, 132.4493) (55.6966, 132.2008) (55.4817, 131.9511) (55.2689, 131.6999) (55.0585, 131.4472) (54.851, 131.1926) (54.6471, 130.936) (54.4469, 130.677) (54.2505, 130.4157) (54.0575, 130.1525) (53.8669, 129.8878) (53.6781, 129.6219) (53.4912, 129.3551) (53.3069, 129.0868) (53.1274, 128.8157) (52.956, 128.5403) (52.8278, 128.3151) (52.7378, 128.1427) (52.6807, 128.0263) (52.6529, 127.9676) knots -1 -1 -1 -1 -1 -1 -0.98571429 -0.97142857 -0.95714286 -0.94285714 -0.92857143 -0.91428571 -0.9 -0.88571429 -0.87142857 -0.85714286 -0.84285714 -0.82857143 -0.81428571 -0.8 -0.78571429 -0.77142857 -0.75714286 -0.74285714 -0.72857143 -0.71428571 -0.7 -0.68571429 -0.67142857 -0.65714286 -0.64285714 -0.62857143 -0.61428571 -0.6 -0.58571429 -0.57142857 -0.55714286 -0.54285714 -0.52857143 -0.51428571 -0.5 -0.48571429 -0.47142857 -0.45714286 -0.44285714 -0.42857143 -0.41428571 -0.4 -0.38571429 -0.37142857 -0.35714286 -0.34285714 -0.32857143 -0.31428571 -0.3 -0.28571429 -0.27142857 -0.25714286 -0.24285714 -0.22857143 -0.21428571 -0.2 -0.18571429 -0.17142857 -0.15714286 -0.14285714 -0.12857143 -0.11428571 -0.1 -0.08571429 -0.07142857 -0.05714286 -0.04285714 -0.02857143 -0.01428571 0 0 0 0 0 0
  line L9 (52.6529, 127.9676) -> (50.7131, 123.8831)
  arc A19 (48.6147, 123.1223) -> (50.7131, 123.8831) centre (49.2791, 124.5641) ccw
  arc A20 (48.6147, 123.1223) -> (38.7127, 127.2239) centre (-8.7656, -1.4025) ccw
  arc A21 (37.7669, 129.2456) -> (38.7127, 127.2239) centre (39.2624, 128.7131) ccw
  line L10 (37.7669, 129.2456) -> (39.2834, 133.5054)
  spline S10 degree 5 poles (39.2834, 133.5054) (39.3052, 133.5666) (39.3472, 133.6893) (39.4054, 133.8748) (39.474, 134.1247) (39.5476, 134.4407) (39.6123, 134.7592) (39.6717, 135.0793) (39.7282, 135.4002) (39.7827, 135.7216) (39.8352, 136.0436) (39.8848, 136.3662) (39.9307, 136.6898) (39.9723, 137.0145) (40.0095, 137.3402) (40.0429, 137.6669) (40.0728, 137.9943) (40.0999, 138.3224) (40.1245, 138.651) (40.1468, 138.9801) (40.1667, 139.3096) (40.1841, 139.6396) (40.1989, 139.9701) (40.211, 140.3012) (40.2205, 140.6328) (40.2274, 140.9648) (40.2319, 141.2973) (40.2341, 141.6302) (40.2341, 141.9635) (40.2319, 142.2971) (40.2275, 142.631) (40.221, 142.9653) (40.2124, 143.2999) (40.2015, 143.6348) (40.1886, 143.97) (40.1736, 144.3055) (40.1565, 144.6413) (40.1374, 144.9774) (40.1163, 145.3137) (40.0933, 145.6502) (40.0684, 145.987) (40.0415, 146.324) (40.0127, 146.6612) (39.9821, 146.9986) (39.9495, 147.3362) (39.9151, 147.674) (39.8789, 148.0119) (39.8408, 148.3501) (39.801, 148.6883) (39.7594, 149.0268) (39.716, 149.3653) (39.6708, 149.704) (39.6239, 150.0429) (39.5753, 150.3818) (39.5249, 150.7209) (39.4729, 151.06) (39.4191, 151.3993) (39.3637, 151.7387) (39.3066, 152.0781) (39.2478, 152.4176) (39.1875, 152.7572) (39.1254, 153.0969) (39.0618, 153.4366) (38.9965, 153.7763) (38.9296, 154.1162) (38.8611, 154.456) (38.7911, 154.7959) (38.7195, 155.1358) (38.6463, 155.4757) (38.5715, 155.8157) (38.4952, 156.1556) (38.4329, 156.4276) (38.3855, 156.6316) (38.3536, 156.7676) (38.3376, 156.8356) knots 0 0 0 0 0 0 0.01428571 0.02857143 0.04285714 0.05714286 0.07142857 0.08571429 0.1 0.11428571 0.12857143 0.14285714 0.15714286 0.17142857 0.18571429 0.2 0.21428571 0.22857143 0.24285714 0.25714286 0.27142857 0.28571429 0.3 0.31428571 0.32857143 0.34285714 0.35714286 0.37142857 0.38571429 0.4 0.41428571 0.42857143 0.44285714 0.45714286 0.47142857 0.48571429 0.5 0.51428571 0.52857143 0.54285714 0.55714286 0.57142857 0.58571429 0.6 0.61428571 0.62857143 0.64285714 0.65714286 0.67142857 0.68571429 0.7 0.71428571 0.72857143 0.74285714 0.75714286 0.77142857 0.78571429 0.8 0.81428571 0.82857143 0.84285714 0.85714286 0.87142857 0.88571429 0.9 0.91428571 0.92857143 0.94285714 0.95714286 0.97142857 0.98571429 1 1 1 1 1 1
  arc A22 (38.3376, 156.8356) -> (29.5609, 159.1873) centre (-8.7656, -1.4025) ccw
  spline S11 degree 5 poles (29.5609, 159.1873) (29.513, 159.1365) (29.4173, 159.0346) (29.2743, 158.8817) (29.0844, 158.6773) (28.8483, 158.421) (28.6136, 158.164) (28.3802, 157.9062) (28.1483, 157.6476) (27.9176, 157.3883) (27.6884, 157.1282) (27.4606, 156.8674) (27.2342, 156.6058) (27.0092, 156.3434) (26.7857, 156.0803) (26.5636, 155.8164) (26.3429, 155.5517) (26.1238, 155.2863) (25.9061, 155.0201) (25.6899, 154.7532) (25.4752, 154.4855) (25.2621, 154.217) (25.0505, 153.9478) (24.8405, 153.6778) (24.632, 153.4071) (24.4251, 153.1356) (24.2199, 152.8633) (24.0162, 152.5903) (23.8142, 152.3165) (23.6139, 152.0419) (23.4152, 151.7666) (23.2182, 151.4905) (23.0229, 151.2136) (22.8294, 150.936) (22.6376, 150.6576) (22.4476, 150.3784) (22.2594, 150.0984) (22.0731, 149.8177) (21.8885, 149.5362) (21.7058, 149.2539) (21.525, 148.9709) (21.3462, 148.6871) (21.1694, 148.4024) (20.9946, 148.117) (20.8218, 147.8307) (20.6511, 147.5437) (20.4824, 147.2559) (20.3158, 146.9673) (20.1512, 146.6779) (19.9889, 146.3878) (19.8288, 146.0967) (19.6712, 145.8048) (19.5162, 145.5121) (19.3637, 145.2184) (19.2138, 144.9239) (19.0663, 144.6286) (18.9211, 144.3325) (18.7781, 144.0356) (18.6375, 143.7379) (18.4997, 143.4393) (18.3652, 143.1398) (18.2346, 142.8391) (18.1083, 142.5371) (17.9862, 142.2339) (17.8679, 141.9297) (17.7523, 141.6246) (17.6388, 141.319) (17.5273, 141.0129) (17.4187, 140.706) (17.3155, 140.3978) (17.2212, 140.0874) (17.1557, 139.8366) (17.1134, 139.6468) (17.0884, 139.5196) (17.0766, 139.4557) knots -1 -1 -1 -1 -1 -1 -0.98571429 -0.97142857 -0.95714286 -0.94285714 -0.92857143 -0.91428571 -0.9 -0.88571429 -0.87142857 -0.85714286 -0.84285714 -0.82857143 -0.81428571 -0.8 -0.78571429 -0.77142857 -0.75714286 -0.74285714 -0.72857143 -0.71428571 -0.7 -0.68571429 -0.67142857 -0.65714286 -0.64285714 -0.62857143 -0.61428571 -0.6 -0.58571429 -0.57142857 -0.55714286 -0.54285714 -0.52857143 -0.51428571 -0.5 -0.48571429 -0.47142857 -0.45714286 -0.44285714 -0.42857143 -0.41428571 -0.4 -0.38571429 -0.37142857 -0.35714286 -0.34285714 -0.32857143 -0.31428571 -0.3 -0.28571429 -0.27142857 -0.25714286 -0.24285714 -0.22857143 -0.21428571 -0.2 -0.18571429 -0.17142857 -0.15714286 -0.14285714 -0.12857143 -0.11428571 -0.1 -0.08571429 -0.07142857 -0.05714286 -0.04285714 -0.02857143 -0.01428571 0 0 0 0 0 0
  line L11 (17.0766, 139.4557) -> (16.2601, 135.0083)
  arc A23 (14.4301, 133.7304) -> (16.2601, 135.0083) centre (14.6987, 135.295) ccw
  arc A24 (14.4301, 133.7304) -> (3.804, 135.1293) centre (-8.7656, -1.4025) ccw
  arc A25 (2.3671, 136.8374) -> (3.804, 135.1293) centre (3.9495, 136.7101) ccw
  line L12 (2.3671, 136.8374) -> (2.7295, 141.3446)
  spline S12 degree 5 poles (2.7295, 141.3446) (2.7347, 141.4093) (2.7434, 141.5387) (2.7516, 141.7329) (2.7533, 141.9921) (2.7425, 142.3163) (2.7227, 142.6408) (2.6972, 142.9653) (2.6687, 143.2899) (2.6382, 143.6144) (2.6055, 143.939) (2.5699, 144.2635) (2.5305, 144.588) (2.4866, 144.9123) (2.4383, 145.2366) (2.386, 145.5608) (2.3301, 145.8848) (2.2713, 146.2087) (2.2101, 146.5325) (2.1464, 146.8561) (2.0804, 147.1796) (2.0118, 147.5028) (1.9406, 147.826) (1.8666, 148.1489) (1.7899, 148.4716) (1.7106, 148.7941) (1.6289, 149.1164) (1.5449, 149.4386) (1.4586, 149.7604) (1.3701, 150.0821) (1.2795, 150.4035) (1.1867, 150.7247) (1.0917, 151.0457) (0.9946, 151.3664) (0.8953, 151.6868) (0.794, 152.007) (0.6906, 152.327) (0.5852, 152.6466) (0.4778, 152.966) (0.3685, 153.2852) (0.2572, 153.604) (0.144, 153.9225) (0.029, 154.2408) (-0.088, 154.5588) (-0.2068, 154.8765) (-0.3275, 155.1938) (-0.4499, 155.5109) (-0.5742, 155.8276) (-0.7002, 156.1441) (-0.828, 156.4602) (-0.9576, 156.776) (-1.0889, 157.0915) (-1.2219, 157.4066) (-1.3566, 157.7214) (-1.493, 158.0359) (-1.631, 158.35) (-1.7708, 158.6638) (-1.9121, 158.9773) (-2.0551, 159.2904) (-2.1997, 159.6031) (-2.346, 159.9155) (-2.4938, 160.2275) (-2.6432, 160.5392) (-2.7942, 160.8505) (-2.9468, 161.1614) (-3.1008, 161.472) (-3.2565, 161.7821) (-3.4136, 162.0919) (-3.5723, 162.4013) (-3.7325, 162.7103) (-3.8942, 163.019) (-4.0248, 163.2656) (-4.1233, 163.4503) (-4.1894, 163.5734) (-4.2224, 163.635) knots 0 0 0 0 0 0 0.01428571 0.02857143 0.04285714 0.05714286 0.07142857 0.08571429 0.1 0.11428571 0.12857143 0.14285714 0.15714286 0.17142857 0.18571429 0.2 0.21428571 0.22857143 0.24285714 0.25714286 0.27142857 0.28571429 0.3 0.31428571 0.32857143 0.34285714 0.35714286 0.37142857 0.38571429 0.4 0.41428571 0.42857143 0.44285714 0.45714286 0.47142857 0.48571429 0.5 0.51428571 0.52857143 0.54285714 0.55714286 0.57142857 0.58571429 0.6 0.61428571 0.62857143 0.64285714 0.65714286 0.67142857 0.68571429 0.7 0.71428571 0.72857143 0.74285714 0.75714286 0.77142857 0.78571429 0.8 0.81428571 0.82857143 0.84285714 0.85714286 0.87142857 0.88571429 0.9 0.91428571 0.92857143 0.94285714 0.95714286 0.97142857 0.98571429 1 1 1 1 1 1
  arc A26 (-4.2224, 163.635) -> (-13.3088, 163.635) centre (-8.7656, -1.4025) ccw